Autodesk Inventor part; units mm, degrees
(part 4 of 16)
  spline S18 degree 3 poles (-31.6012, 101.0382) (-31.4716, 101.001) (-31.3425, 100.9618) (-31.2141, 100.9205) (-31.1447, 100.8982) (-31.0755, 100.8753) (-31.0064, 100.8518) (-30.9411, 100.8296) (-30.876, 100.8067) (-30.8111, 100.7833) (-30.7498, 100.7612) (-30.6887, 100.7385) (-30.6278, 100.7153) (-30.5706, 100.6935) (-30.5136, 100.6712) (-30.4567, 100.6484) (-30.4035, 100.627) (-30.3504, 100.6052) (-30.2976, 100.5829) (-30.2483, 100.5621) (-30.1992, 100.5408) (-30.1504, 100.5192) (-30.105, 100.4991) (-30.0599, 100.4786) (-30.0149, 100.4577) (-29.9734, 100.4384) (-29.9322, 100.4188) (-29.8911, 100.3988) (-29.8535, 100.3805) (-29.816, 100.3618) (-29.7787, 100.3429) (-29.7449, 100.3257) (-29.7113, 100.3082) (-29.6778, 100.2904) (-29.6477, 100.2744) (-29.6178, 100.2582) (-29.588, 100.2417) (-29.5487, 100.2198) (-29.5097, 100.1974) (-29.4708, 100.1747) (-29.4621, 100.1696) (-29.4535, 100.1645) (-29.4447, 100.1595) (-29.4362, 100.1546) (-29.4276, 100.1498) (-29.419, 100.1451) (-29.4105, 100.1404) (-29.4021, 100.1359) (-29.3935, 100.1314) (-29.3852, 100.127) (-29.3768, 100.1227) (-29.3684, 100.1184) (-29.3601, 100.1143) (-29.3518, 100.1102) (-29.3434, 100.1062) (-29.3352, 100.1023) (-29.3269, 100.0984) (-29.3186, 100.0947) (-29.3104, 100.091) (-29.3021, 100.0874) (-29.2938, 100.0839) (-29.2856, 100.0804) (-29.2774, 100.077) (-29.2691, 100.0737) (-29.2608, 100.0705) (-29.2525, 100.0674) (-29.2441, 100.0643) (-29.2357, 100.0613) (-29.2273, 100.0584) (-29.2189, 100.0556) (-29.2103, 100.0528) (-29.2017, 100.0501) (-29.1931, 100.0476) (-29.1843, 100.0451) (-29.1755, 100.0427) (-29.1666, 100.0404) (-29.1575, 100.0381) (-29.1483, 100.036) (-29.1391, 100.0341) (-29.1295, 100.0321) (-29.1199, 100.0303) (-29.1102, 100.0288) (-29.1, 100.0271) (-29.0898, 100.0257) (-29.0795, 100.0246) (-29.0685, 100.0235) (-29.0574, 100.0226) (-29.0464, 100.0221) (-29.0343, 100.0216) (-29.0223, 100.0214) (-29.0103, 100.0217) (-28.997, 100.0221) (-28.9837, 100.0229) (-28.9705, 100.0243) (-28.9558, 100.0259) (-28.9412, 100.0282) (-28.9266, 100.0312) (-28.9103, 100.0345) (-28.8942, 100.0387) (-28.8783, 100.0439) (-28.8605, 100.0497) (-28.8431, 100.0566) (-28.8262, 100.0646) (-28.8074, 100.0735) (-28.7893, 100.0838) (-28.7719, 100.0953) (-28.7531, 100.1078) (-28.7353, 100.1218) (-28.7189, 100.1373) (-28.7032, 100.1521) (-28.6889, 100.1682) (-28.6748, 100.1845) (-28.6053, 100.2653) (-28.5428, 100.3517) (-28.4763, 100.4349) (-28.4098, 100.518) (-28.3392, 100.5979) (-28.2756, 100.6835) (-28.2628, 100.7008) (-28.2502, 100.7183) (-28.2392, 100.7368) (-28.2277, 100.7562) (-28.218, 100.7767) (-28.2099, 100.7978) (-28.2024, 100.8172) (-28.1964, 100.8372) (-28.1918, 100.8574) (-28.1877, 100.8757) (-28.1848, 100.8942) (-28.183, 100.9129) (-28.1815, 100.9295) (-28.1809, 100.9461) (-28.1812, 100.9628) (-28.1815, 100.9776) (-28.1825, 100.9924) (-28.1842, 101.0071) (-28.1857, 101.0203) (-28.1878, 101.0334) (-28.1904, 101.0464) (-28.1927, 101.0582) (-28.1955, 101.07) (-28.1987, 101.0816) (-28.2016, 101.0923) (-28.2048, 101.1028) (-28.2084, 101.1133) (-28.2117, 101.1231) (-28.2153, 101.1328) (-28.2192, 101.1424) (-28.2228, 101.1515) (-28.2266, 101.1605) (-28.2307, 101.1694) (-28.2346, 101.178) (-28.2387, 101.1865) (-28.2429, 101.1949) (-28.247, 101.2031) (-28.2513, 101.2112) (-28.2558, 101.2192) (-28.2601, 101.227) (-28.2646, 101.2348) (-28.2692, 101.2425) (-28.2738, 101.2502) (-28.2784, 101.2578) (-28.2832, 101.2653) (-28.288, 101.2727) (-28.2929, 101.2802) (-28.2979, 101.2875) (-28.3029, 101.2949) (-28.308, 101.3022) (-28.3132, 101.3095) (-28.3185, 101.3168) (-28.3238, 101.3241) (-28.3292, 101.3313) (-28.3347, 101.3385) (-28.3402, 101.3458) (-28.3459, 101.3529) (-28.3516, 101.3602) (-28.3574, 101.3674) (-28.3633, 101.3746) (-28.3693, 101.3819) (-28.3753, 101.3891) (-28.3814, 101.3963) (-28.3877, 101.4037) (-28.394, 101.4109) (-28.4004, 101.4181) (-28.4069, 101.4255) (-28.4134, 101.4329) (-28.4201, 101.4401) (-28.4269, 101.4475) (-28.4338, 101.4549) (-28.4406, 101.4622) (-28.4713, 101.4951) (-28.5017, 101.5283) (-28.5317, 101.5619) (-28.5544, 101.5873) (-28.5767, 101.6129) (-28.5989, 101.6388) (-28.6236, 101.6675) (-28.6481, 101.6965) (-28.6723, 101.7258) (-28.699, 101.758) (-28.7254, 101.7904) (-28.7515, 101.8231) (-28.78, 101.8588) (-28.8082, 101.8948) (-28.8361, 101.931) (-28.8663, 101.9703) (-28.8962, 102.0098) (-28.9258, 102.0496) (-28.9577, 102.0926) (-28.9892, 102.1358) (-29.0203, 102.1793) (-29.0536, 102.226) (-29.0866, 102.2729) (-29.1191, 102.3202) (-29.1538, 102.3706) (-29.1881, 102.4214) (-29.222, 102.4724) (-29.2579, 102.5267) (-29.2934, 102.5814) (-29.3284, 102.6363) (-29.3655, 102.6945) (-29.4021, 102.753) (-29.4382, 102.8119) (-29.4763, 102.8741) (-29.5138, 102.9366) (-29.5508, 102.9994) (-29.6192, 103.1156) (-29.6857, 103.233) (-29.7505, 103.3512) knots 0 0 0 0 0.057795 0.057795 0.057795 0.089038 0.089038 0.089038 0.118617 0.118617 0.118617 0.14653 0.14653 0.14653 0.172778 0.172778 0.172778 0.19736 0.19736 0.19736 0.220277 0.220277 0.220277 0.241529 0.241529 0.241529 0.261115 0.261115 0.261115 0.279036 0.279036 0.279036 0.295292 0.295292 0.295292 0.309882 0.309882 0.309882 0.329164 0.329164 0.329164 0.333477 0.333477 0.333477 0.337694 0.337694 0.337694 0.34182 0.34182 0.34182 0.345864 0.345864 0.345864 0.349834 0.349834 0.349834 0.353742 0.353742 0.353742 0.3576 0.3576 0.3576 0.361424 0.361424 0.361424 0.365232 0.365232 0.365232 0.369048 0.369048 0.369048 0.372899 0.372899 0.372899 0.376819 0.376819 0.376819 0.380853 0.380853 0.380853 0.385052 0.385052 0.385052 0.389482 0.389482 0.389482 0.394225 0.394225 0.394225 0.399381 0.399381 0.399381 0.405067 0.405067 0.405067 0.411413 0.411413 0.411413 0.418548 0.418548 0.418548 0.426565 0.426565 0.426565 0.435472 0.435472 0.435472 0.445133 0.445133 0.445133 0.45436 0.45436 0.45436 0.5 0.5 0.5 0.54564 0.54564 0.54564 0.554867 0.554867 0.554867 0.564528 0.564528 0.564528 0.573435 0.573435 0.573435 0.581452 0.581452 0.581452 0.588587 0.588587 0.588587 0.594933 0.594933 0.594933 0.600619 0.600619 0.600619 0.605775 0.605775 0.605775 0.610518 0.610518 0.610518 0.614948 0.614948 0.614948 0.619147 0.619147 0.619147 0.623181 0.623181 0.623181 0.627101 0.627101 0.627101 0.630952 0.630952 0.630952 0.634768 0.634768 0.634768 0.638576 0.638576 0.638576 0.6424 0.6424 0.6424 0.646258 0.646258 0.646258 0.650166 0.650166 0.650166 0.654136 0.654136 0.654136 0.65818 0.65818 0.65818 0.662306 0.662306 0.662306 0.666523 0.666523 0.666523 0.670836 0.670836 0.670836 0.690118 0.690118 0.690118 0.704708 0.704708 0.704708 0.720964 0.720964 0.720964 0.738885 0.738885 0.738885 0.758471 0.758471 0.758471 0.779723 0.779723 0.779723 0.80264 0.80264 0.80264 0.827222 0.827222 0.827222 0.85347 0.85347 0.85347 0.881383 0.881383 0.881383 0.910962 0.910962 0.910962 0.942205 0.942205 0.942205 1 1 1 1
  arc A220 (-31.6012, 101.0382) -> (-32.2774, 100.0959) centre (0.0435, 77.6158) ccw
  spline S19 degree 3 poles (-33.8761, 97.6022) (-33.7433, 97.5786) (-33.6109, 97.5531) (-33.4789, 97.5256) (-33.4075, 97.5106) (-33.3363, 97.4951) (-33.2652, 97.4789) (-33.1979, 97.4636) (-33.1307, 97.4477) (-33.0637, 97.4312) (-33.0004, 97.4156) (-32.9373, 97.3995) (-32.8744, 97.3828) (-32.8152, 97.3671) (-32.7561, 97.3509) (-32.6972, 97.3341) (-32.642, 97.3184) (-32.587, 97.3022) (-32.5321, 97.2856) (-32.4809, 97.27) (-32.4299, 97.254) (-32.379, 97.2376) (-32.3318, 97.2223) (-32.2848, 97.2067) (-32.2379, 97.1906) (-32.1946, 97.1757) (-32.1515, 97.1605) (-32.1086, 97.1449) (-32.0692, 97.1307) (-32.0301, 97.1161) (-31.991, 97.1011) (-31.9556, 97.0875) (-31.9203, 97.0736) (-31.8851, 97.0594) (-31.8535, 97.0467) (-31.8221, 97.0337) (-31.7907, 97.0204) (-31.7493, 97.0028) (-31.7082, 96.9845) (-31.6672, 96.966) (-31.658, 96.9619) (-31.6489, 96.9577) (-31.6396, 96.9536) (-31.6306, 96.9497) (-31.6216, 96.9458) (-31.6125, 96.942) (-31.6036, 96.9382) (-31.5947, 96.9346) (-31.5858, 96.931) (-31.577, 96.9275) (-31.5682, 96.9241) (-31.5594, 96.9208) (-31.5507, 96.9175) (-31.542, 96.9143) (-31.5333, 96.9112) (-31.5247, 96.9082) (-31.5161, 96.9052) (-31.5074, 96.9024) (-31.4989, 96.8995) (-31.4903, 96.8968) (-31.4817, 96.8942) (-31.4731, 96.8916) (-31.4646, 96.8891) (-31.456, 96.8867) (-31.4474, 96.8844) (-31.4388, 96.8821) (-31.4302, 96.88) (-31.4215, 96.8778) (-31.4129, 96.8758) (-31.4042, 96.8739) (-31.3954, 96.872) (-31.3866, 96.8703) (-31.3777, 96.8687) (-31.3687, 96.8671) (-31.3597, 96.8656) (-31.3506, 96.8643) (-31.3413, 96.863) (-31.332, 96.8618) (-31.3226, 96.8609) (-31.3129, 96.8599) (-31.3031, 96.8591) (-31.2933, 96.8586) (-31.283, 96.858) (-31.2726, 96.8577) (-31.2623, 96.8577) (-31.2512, 96.8577) (-31.2402, 96.858) (-31.2291, 96.8587) (-31.2171, 96.8594) (-31.2051, 96.8605) (-31.1932, 96.8621) (-31.18, 96.8638) (-31.1669, 96.866) (-31.1539, 96.8688) (-31.1395, 96.8719) (-31.1251, 96.8757) (-31.111, 96.8802) (-31.0951, 96.8852) (-31.0795, 96.8911) (-31.0643, 96.8979) (-31.0472, 96.9055) (-31.0306, 96.9142) (-31.0146, 96.9239) (-30.9968, 96.9347) (-30.9799, 96.9469) (-30.9638, 96.9602) (-30.9465, 96.9746) (-30.9302, 96.9903) (-30.9155, 97.0074) (-30.9014, 97.0238) (-30.8889, 97.0413) (-30.8766, 97.059) (-30.8159, 97.1467) (-30.7628, 97.2391) (-30.7053, 97.3287) (-30.6479, 97.4184) (-30.586, 97.5052) (-30.5317, 97.5969) (-30.5207, 97.6155) (-30.5101, 97.6343) (-30.5011, 97.6538) (-30.4917, 97.6743) (-30.4841, 97.6957) (-30.4783, 97.7175) (-30.4729, 97.7376) (-30.469, 97.7581) (-30.4665, 97.7787) (-30.4644, 97.7973) (-30.4634, 97.8161) (-30.4636, 97.8348) (-30.4638, 97.8514) (-30.465, 97.8681) (-30.467, 97.8846) (-30.4689, 97.8993) (-30.4714, 97.9139) (-30.4746, 97.9284) (-30.4775, 97.9413) (-30.481, 97.9542) (-30.4849, 97.9668) (-30.4885, 97.9783) (-30.4924, 97.9897) (-30.4968, 98.0009) (-30.5008, 98.0112) (-30.5052, 98.0214) (-30.5098, 98.0315) (-30.5141, 98.0409) (-30.5187, 98.0501) (-30.5235, 98.0593) (-30.5281, 98.068) (-30.5329, 98.0765) (-30.5378, 98.085) (-30.5426, 98.0931) (-30.5476, 98.1011) (-30.5527, 98.109) (-30.5576, 98.1167) (-30.5627, 98.1243) (-30.568, 98.1318) (-30.5731, 98.1392) (-30.5784, 98.1464) (-30.5838, 98.1536) (-30.5891, 98.1607) (-30.5946, 98.1678) (-30.6001, 98.1748) (-30.6056, 98.1817) (-30.6113, 98.1886) (-30.617, 98.1954) (-30.6228, 98.2022) (-30.6286, 98.2089) (-30.6345, 98.2156) (-30.6405, 98.2223) (-30.6466, 98.229) (-30.6527, 98.2356) (-30.6589, 98.2423) (-30.6652, 98.2489) (-30.6716, 98.2554) (-30.678, 98.262) (-30.6845, 98.2686) (-30.6911, 98.2751) (-30.6978, 98.2818) (-30.7046, 98.2883) (-30.7115, 98.2948) (-30.7184, 98.3015) (-30.7255, 98.308) (-30.7326, 98.3146) (-30.7398, 98.3212) (-30.7471, 98.3278) (-30.7545, 98.3343) (-30.762, 98.341) (-30.7696, 98.3476) (-30.7772, 98.3542) (-30.8112, 98.3837) (-30.8449, 98.4135) (-30.8782, 98.4438) (-30.9034, 98.4667) (-30.9283, 98.4898) (-30.9531, 98.5132) (-30.9807, 98.5393) (-31.008, 98.5655) (-31.0352, 98.5921) (-31.0651, 98.6213) (-31.0947, 98.6508) (-31.1241, 98.6806) (-31.1562, 98.7131) (-31.188, 98.7459) (-31.2195, 98.779) (-31.2537, 98.8149) (-31.2876, 98.8512) (-31.3211, 98.8877) (-31.3573, 98.927) (-31.3932, 98.9667) (-31.4286, 99.0068) (-31.4667, 99.0497) (-31.5044, 99.0929) (-31.5417, 99.1365) (-31.5815, 99.1831) (-31.6209, 99.23) (-31.6599, 99.2772) (-31.7013, 99.3274) (-31.7423, 99.3781) (-31.7829, 99.429) (-31.8259, 99.483) (-31.8684, 99.5374) (-31.9104, 99.5922) (-31.9548, 99.65) (-31.9986, 99.7083) (-32.0419, 99.7669) (-32.1221, 99.8754) (-32.2006, 99.9851) (-32.2774, 100.0959) knots 0 0 0 0 0.057795 0.057795 0.057795 0.089038 0.089038 0.089038 0.118617 0.118617 0.118617 0.14653 0.14653 0.14653 0.172778 0.172778 0.172778 0.19736 0.19736 0.19736 0.220277 0.220277 0.220277 0.241529 0.241529 0.241529 0.261115 0.261115 0.261115 0.279036 0.279036 0.279036 0.295292 0.295292 0.295292 0.309882 0.309882 0.309882 0.329164 0.329164 0.329164 0.333477 0.333477 0.333477 0.337694 0.337694 0.337694 0.34182 0.34182 0.34182 0.345864 0.345864 0.345864 0.349834 0.349834 0.349834 0.353742 0.353742 0.353742 0.3576 0.3576 0.3576 0.361424 0.361424 0.361424 0.365232 0.365232 0.365232 0.369048 0.369048 0.369048 0.372899 0.372899 0.372899 0.376819 0.376819 0.376819 0.380853 0.380853 0.380853 0.385052 0.385052 0.385052 0.389482 0.389482 0.389482 0.394225 0.394225 0.394225 0.399381 0.399381 0.399381 0.405067 0.405067 0.405067 0.411413 0.411413 0.411413 0.418548 0.418548 0.418548 0.426565 0.426565 0.426565 0.435472 0.435472 0.435472 0.445133 0.445133 0.445133 0.45436 0.45436 0.45436 0.5 0.5 0.5 0.54564 0.54564 0.54564 0.554867 0.554867 0.554867 0.564528 0.564528 0.564528 0.573435 0.573435 0.573435 0.581452 0.581452 0.581452 0.588587 0.588587 0.588587 0.594933 0.594933 0.594933 0.600619 0.600619 0.600619 0.605775 0.605775 0.605775 0.610518 0.610518 0.610518 0.614948 0.614948 0.614948 0.619147 0.619147 0.619147 0.623181 0.623181 0.623181 0.627101 0.627101 0.627101 0.630952 0.630952 0.630952 0.634768 0.634768 0.634768 0.638576 0.638576 0.638576 0.6424 0.6424 0.6424 0.646258 0.646258 0.646258 0.650166 0.650166 0.650166 0.654136 0.654136 0.654136 0.65818 0.65818 0.65818 0.662306 0.662306 0.662306 0.666523 0.666523 0.666523 0.670836 0.670836 0.670836 0.690118 0.690118 0.690118 0.704708 0.704708 0.704708 0.720964 0.720964 0.720964 0.738885 0.738885 0.738885 0.758471 0.758471 0.758471 0.779723 0.779723 0.779723 0.80264 0.80264 0.80264 0.827222 0.827222 0.827222 0.85347 0.85347 0.85347 0.881383 0.881383 0.881383 0.910962 0.910962 0.910962 0.942205 0.942205 0.942205 1 1 1 1
  arc A221 (-33.8761, 97.6022) -> (-34.4501, 96.5943) centre (0.0435, 77.6158) ccw
  spline S20 degree 3 poles (-35.7795, 93.9471) (-35.6449, 93.9376) (-35.5105, 93.9261) (-35.3764, 93.9124) (-35.3038, 93.9051) (-35.2314, 93.8971) (-35.159, 93.8884) (-35.0904, 93.8802) (-35.022, 93.8714) (-34.9536, 93.862) (-34.8891, 93.8531) (-34.8246, 93.8437) (-34.7603, 93.8336) (-34.6997, 93.8242) (-34.6393, 93.8143) (-34.579, 93.8037) (-34.5225, 93.7939) (-34.466, 93.7836) (-34.4097, 93.7727) (-34.3572, 93.7626) (-34.3048, 93.7521) (-34.2524, 93.741) (-34.2039, 93.7308) (-34.1555, 93.7201) (-34.1071, 93.709) (-34.0626, 93.6988) (-34.0181, 93.6882) (-33.9738, 93.6772) (-33.9332, 93.6671) (-33.8927, 93.6566) (-33.8523, 93.6458) (-33.8156, 93.636) (-33.7791, 93.6259) (-33.7426, 93.6155) (-33.7099, 93.6061) (-33.6772, 93.5965) (-33.6447, 93.5865) (-33.6017, 93.5733) (-33.5588, 93.5595) (-33.5161, 93.5453) (-33.5066, 93.5422) (-33.497, 93.539) (-33.4874, 93.5359) (-33.4781, 93.5329) (-33.4687, 93.53) (-33.4593, 93.5271) (-33.45, 93.5244) (-33.4408, 93.5217) (-33.4315, 93.5191) (-33.4224, 93.5165) (-33.4133, 93.514) (-33.4042, 93.5116) (-33.3952, 93.5093) (-33.3863, 93.507) (-33.3772, 93.5049) (-33.3684, 93.5027) (-33.3595, 93.5007) (-33.3506, 93.4987) (-33.3418, 93.4968) (-33.333, 93.495) (-33.3241, 93.4933) (-33.3154, 93.4916) (-33.3066, 93.49) (-33.2978, 93.4886) (-33.289, 93.4871) (-33.2802, 93.4858) (-33.2714, 93.4845) (-33.2626, 93.4833) (-33.2538, 93.4822) (-33.2449, 93.4813) (-33.236, 93.4803) (-33.227, 93.4795) (-33.2181, 93.4788) (-33.2089, 93.4781) (-33.1998, 93.4776) (-33.1907, 93.4773) (-33.1813, 93.4769) (-33.1718, 93.4768) (-33.1624, 93.4768) (-33.1526, 93.4768) (-33.1428, 93.4771) (-33.1331, 93.4776) (-33.1227, 93.4781) (-33.1124, 93.4789) (-33.1021, 93.48) (-33.0911, 93.4811) (-33.0801, 93.4826) (-33.0692, 93.4844) (-33.0573, 93.4863) (-33.0455, 93.4887) (-33.0338, 93.4915) (-33.0209, 93.4946) (-33.0081, 93.4982) (-32.9955, 93.5023) (-32.9814, 93.5069) (-32.9676, 93.5122) (-32.954, 93.5181) (-32.9387, 93.5248) (-32.9238, 93.5323) (-32.9094, 93.5406) (-32.8932, 93.5499) (-32.8776, 93.5603) (-32.8627, 93.5717) (-32.8462, 93.5843) (-32.8306, 93.5981) (-32.816, 93.613) (-32.8002, 93.6292) (-32.7857, 93.6466) (-32.7729, 93.6651) (-32.7606, 93.6828) (-32.7499, 93.7016) (-32.7396, 93.7205) (-32.6884, 93.814) (-32.6452, 93.9115) (-32.5974, 94.0066) (-32.5497, 94.1018) (-32.4972, 94.1946) (-32.4528, 94.2915) (-32.4438, 94.3111) (-32.4352, 94.3309) (-32.4283, 94.3513) (-32.4211, 94.3726) (-32.4158, 94.3947) (-32.4123, 94.417) (-32.409, 94.4375) (-32.4073, 94.4583) (-32.407, 94.4791) (-32.4068, 94.4978) (-32.4078, 94.5166) (-32.41, 94.5352) (-32.4119, 94.5517) (-32.4148, 94.5681) (-32.4186, 94.5844) (-32.4219, 94.5988) (-32.426, 94.6131) (-32.4307, 94.6271) (-32.4349, 94.6397) (-32.4397, 94.6521) (-32.4449, 94.6643) (-32.4497, 94.6753) (-32.4548, 94.6862) (-32.4603, 94.6969) (-32.4654, 94.7068) (-32.4708, 94.7164) (-32.4764, 94.7259) (-32.4817, 94.7348) (-32.4873, 94.7436) (-32.493, 94.7522) (-32.4985, 94.7603) (-32.5041, 94.7683) (-32.5099, 94.7762) (-32.5155, 94.7838) (-32.5213, 94.7912) (-32.5272, 94.7986) (-32.5329, 94.8057) (-32.5388, 94.8127) (-32.5448, 94.8196) (-32.5507, 94.8264) (-32.5567, 94.8331) (-32.5628, 94.8397) (-32.5688, 94.8462) (-32.575, 94.8527) (-32.5812, 94.859) (-32.5875, 94.8653) (-32.5938, 94.8716) (-32.6002, 94.8777) (-32.6066, 94.8839) (-32.6132, 94.89) (-32.6197, 94.896) (-32.6264, 94.9021) (-32.6331, 94.9081) (-32.6399, 94.914) (-32.6468, 94.92) (-32.6537, 94.9259) (-32.6607, 94.9317) (-32.6678, 94.9377) (-32.675, 94.9435) (-32.6823, 94.9493) (-32.6896, 94.9552) (-32.6971, 94.961) (-32.7045, 94.9668) (-32.7122, 94.9727) (-32.7199, 94.9785) (-32.7276, 94.9842) (-32.7355, 94.9901) (-32.7434, 94.9959) (-32.7514, 95.0016) (-32.7596, 95.0074) (-32.7679, 95.0132) (-32.7761, 95.019) (-32.813, 95.0448) (-32.8497, 95.0709) (-32.8859, 95.0975) (-32.9134, 95.1176) (-32.9406, 95.1381) (-32.9677, 95.1587) (-32.9978, 95.1817) (-33.0278, 95.205) (-33.0575, 95.2285) (-33.0903, 95.2545) (-33.1229, 95.2808) (-33.1552, 95.3073) (-33.1905, 95.3363) (-33.2256, 95.3656) (-33.2604, 95.3952) (-33.2982, 95.4274) (-33.3356, 95.4598) (-33.3728, 95.4926) (-33.4129, 95.528) (-33.4527, 95.5638) (-33.4922, 95.5998) (-33.5345, 95.6385) (-33.5765, 95.6776) (-33.6182, 95.7171) (-33.6626, 95.7592) (-33.7067, 95.8017) (-33.7504, 95.8446) (-33.7969, 95.8903) (-33.843, 95.9363) (-33.8886, 95.9828) (-33.937, 96.032) (-33.985, 96.0816) (-34.0325, 96.1317) (-34.0827, 96.1846) (-34.1324, 96.238) (-34.1816, 96.2917) (-34.2727, 96.3912) (-34.3622, 96.4921) (-34.4501, 96.5943) knots 0 0 0 0 0.057795 0.057795 0.057795 0.089038 0.089038 0.089038 0.118617 0.118617 0.118617 0.14653 0.14653 0.14653 0.172778 0.172778 0.172778 0.19736 0.19736 0.19736 0.220277 0.220277 0.220277 0.241529 0.241529 0.241529 0.261115 0.261115 0.261115 0.279036 0.279036 0.279036 0.295292 0.295292 0.295292 0.309882 0.309882 0.309882 0.329164 0.329164 0.329164 0.333477 0.333477 0.333477 0.337694 0.337694 0.337694 0.34182 0.34182 0.34182 0.345864 0.345864 0.345864 0.349834 0.349834 0.349834 0.353742 0.353742 0.353742 0.3576 0.3576 0.3576 0.361424 0.361424 0.361424 0.365232 0.365232 0.365232 0.369048 0.369048 0.369048 0.372899 0.372899 0.372899 0.376819 0.376819 0.376819 0.380853 0.380853 0.380853 0.385052 0.385052 0.385052 0.389482 0.389482 0.389482 0.394225 0.394225 0.394225 0.399381 0.399381 0.399381 0.405067 0.405067 0.405067 0.411413 0.411413 0.411413 0.418548 0.418548 0.418548 0.426565 0.426565 0.426565 0.435472 0.435472 0.435472 0.445133 0.445133 0.445133 0.45436 0.45436 0.45436 0.5 0.5 0.5 0.54564 0.54564 0.54564 0.554867 0.554867 0.554867 0.564528 0.564528 0.564528 0.573435 0.573435 0.573435 0.581452 0.581452 0.581452 0.588587 0.588587 0.588587 0.594933 0.594933 0.594933 0.600619 0.600619 0.600619 0.605775 0.605775 0.605775 0.610518 0.610518 0.610518 0.614948 0.614948 0.614948 0.619147 0.619147 0.619147 0.623181 0.623181 0.623181 0.627101 0.627101 0.627101 0.630952 0.630952 0.630952 0.634768 0.634768 0.634768 0.638576 0.638576 0.638576 0.6424 0.6424 0.6424 0.646258 0.646258 0.646258 0.650166 0.650166 0.650166 0.654136 0.654136 0.654136 0.65818 0.65818 0.65818 0.662306 0.662306 0.662306 0.666523 0.666523 0.666523 0.670836 0.670836 0.670836 0.690118 0.690118 0.690118 0.704708 0.704708 0.704708 0.720964 0.720964 0.720964 0.738885 0.738885 0.738885 0.758471 0.758471 0.758471 0.779723 0.779723 0.779723 0.80264 0.80264 0.80264 0.827222 0.827222 0.827222 0.85347 0.85347 0.85347 0.881383 0.881383 0.881383 0.910962 0.910962 0.910962 0.942205 0.942205 0.942205 1 1 1 1
  arc A222 (-35.7795, 93.9471) -> (-36.245, 92.8848) centre (0.0435, 77.6158) ccw
  spline S21 degree 3 poles (-37.2903, 90.1131) (-37.1555, 90.1177) (-37.0207, 90.1203) (-36.8858, 90.1208) (-36.8129, 90.121) (-36.74, 90.1207) (-36.6671, 90.1196) (-36.5981, 90.1186) (-36.5291, 90.117) (-36.4601, 90.1148) (-36.395, 90.1127) (-36.3299, 90.1101) (-36.2648, 90.1068) (-36.2037, 90.1038) (-36.1425, 90.1002) (-36.0814, 90.096) (-36.0242, 90.0921) (-35.967, 90.0878) (-35.9098, 90.0829) (-35.8565, 90.0783) (-35.8033, 90.0733) (-35.7501, 90.0678) (-35.7008, 90.0627) (-35.6515, 90.0571) (-35.6023, 90.0511) (-35.5569, 90.0456) (-35.5116, 90.0397) (-35.4663, 90.0334) (-35.4249, 90.0276) (-35.3835, 90.0215) (-35.3422, 90.015) (-35.3047, 90.009) (-35.2673, 90.0028) (-35.23, 89.9962) (-35.1964, 89.9903) (-35.1629, 89.9842) (-35.1295, 89.9776) (-35.0854, 89.969) (-35.0413, 89.9597) (-34.9974, 89.9501) (-34.9875, 89.948) (-34.9777, 89.9458) (-34.9679, 89.9438) (-34.9582, 89.9417) (-34.9486, 89.9398) (-34.9389, 89.938) (-34.9295, 89.9362) (-34.92, 89.9345) (-34.9105, 89.9328) (-34.9012, 89.9312) (-34.8919, 89.9297) (-34.8825, 89.9283) (-34.8734, 89.9269) (-34.8642, 89.9256) (-34.855, 89.9244) (-34.846, 89.9232) (-34.8369, 89.9221) (-34.8279, 89.9211) (-34.8189, 89.9201) (-34.81, 89.9192) (-34.801, 89.9185) (-34.7921, 89.9177) (-34.7832, 89.917) (-34.7743, 89.9165) (-34.7654, 89.916) (-34.7565, 89.9155) (-34.7477, 89.9152) (-34.7388, 89.915) (-34.7299, 89.9148) (-34.721, 89.9148) (-34.712, 89.9147) (-34.703, 89.9149) (-34.694, 89.9151) (-34.6849, 89.9154) (-34.6757, 89.9158) (-34.6666, 89.9165) (-34.6572, 89.9171) (-34.6478, 89.9179) (-34.6385, 89.9189) (-34.6287, 89.92) (-34.619, 89.9213) (-34.6093, 89.9228) (-34.5991, 89.9244) (-34.5889, 89.9263) (-34.5788, 89.9284) (-34.568, 89.9307) (-34.5572, 89.9333) (-34.5465, 89.9362) (-34.5349, 89.9394) (-34.5235, 89.943) (-34.5121, 89.947) (-34.4996, 89.9514) (-34.4872, 89.9563) (-34.4751, 89.9618) (-34.4616, 89.9678) (-34.4484, 89.9745) (-34.4355, 89.9818) (-34.421, 89.99) (-34.407, 89.999) (-34.3935, 90.0088) (-34.3783, 90.0198) (-34.3639, 90.0318) (-34.3503, 90.0446) (-34.3351, 90.0589) (-34.3211, 90.0743) (-34.3082, 90.0906) (-34.2942, 90.1084) (-34.2815, 90.1272) (-34.2707, 90.1469) (-34.2604, 90.1658) (-34.2517, 90.1856) (-34.2434, 90.2055) (-34.2022, 90.3038) (-34.1695, 90.4053) (-34.1319, 90.5049) (-34.0944, 90.6045) (-34.0519, 90.7023) (-34.0179, 90.8034) (-34.011, 90.8238) (-34.0045, 90.8444) (-33.9998, 90.8654) (-33.9948, 90.8874) (-33.9919, 90.9098) (-33.9907, 90.9324) (-33.9896, 90.9532) (-33.99, 90.974) (-33.9919, 90.9947) (-33.9937, 91.0134) (-33.9966, 91.0319) (-34.0007, 91.0502) (-34.0044, 91.0664) (-34.009, 91.0825) (-34.0144, 91.0982) (-34.0193, 91.1122) (-34.0248, 91.126) (-34.031, 91.1394) (-34.0365, 91.1515) (-34.0425, 91.1633) (-34.049, 91.1749) (-34.0549, 91.1854) (-34.0611, 91.1957) (-34.0677, 91.2058) (-34.0738, 91.215) (-34.0802, 91.2241) (-34.0868, 91.233) (-34.093, 91.2412) (-34.0994, 91.2494) (-34.106, 91.2573) (-34.1123, 91.2648) (-34.1187, 91.2722) (-34.1253, 91.2794) (-34.1317, 91.2864) (-34.1382, 91.2932) (-34.1448, 91.2999) (-34.1513, 91.3064) (-34.1579, 91.3127) (-34.1645, 91.319) (-34.1711, 91.3251) (-34.1778, 91.3311) (-34.1845, 91.3371) (-34.1912, 91.3429) (-34.198, 91.3487) (-34.2049, 91.3543) (-34.2118, 91.36) (-34.2187, 91.3655) (-34.2257, 91.371) (-34.2328, 91.3764) (-34.2399, 91.3818) (-34.2471, 91.3871) (-34.2543, 91.3925) (-34.2617, 91.3977) (-34.269, 91.4029) (-34.2765, 91.4081) (-34.284, 91.4133) (-34.2916, 91.4184) (-34.2993, 91.4235) (-34.307, 91.4286) (-34.3148, 91.4336) (-34.3228, 91.4387) (-34.3308, 91.4437) (-34.3388, 91.4486) (-34.347, 91.4537) (-34.3553, 91.4586) (-34.3636, 91.4635) (-34.372, 91.4685) (-34.3805, 91.4735) (-34.3891, 91.4783) (-34.3979, 91.4833) (-34.4067, 91.4882) (-34.4155, 91.493) (-34.4548, 91.5148) (-34.494, 91.537) (-34.5329, 91.5596) (-34.5623, 91.5768) (-34.5915, 91.5943) (-34.6206, 91.612) (-34.653, 91.6317) (-34.6852, 91.6518) (-34.7172, 91.6721) (-34.7526, 91.6944) (-34.7877, 91.7172) (-34.8226, 91.7402) (-34.8608, 91.7653) (-34.8987, 91.7908) (-34.9364, 91.8166) (-34.9773, 91.8446) (-35.018, 91.873) (-35.0584, 91.9018) (-35.102, 91.9327) (-35.1453, 91.9641) (-35.1883, 91.9959) (-35.2345, 92.03) (-35.2803, 92.0644) (-35.3259, 92.0993) (-35.3745, 92.1366) (-35.4228, 92.1743) (-35.4707, 92.2124) (-35.5217, 92.2529) (-35.5724, 92.2939) (-35.6226, 92.3353) (-35.6759, 92.3792) (-35.7288, 92.4235) (-35.7813, 92.4684) (-35.8367, 92.5157) (-35.8917, 92.5636) (-35.9463, 92.6119) (-36.0473, 92.7013) (-36.1468, 92.7924) (-36.245, 92.8848) knots 0 0 0 0 0.057795 0.057795 0.057795 0.089038 0.089038 0.089038 0.118617 0.118617 0.118617 0.14653 0.14653 0.14653 0.172778 0.172778 0.172778 0.19736 0.19736 0.19736 0.220277 0.220277 0.220277 0.241529 0.241529 0.241529 0.261115 0.261115 0.261115 0.279036 0.279036 0.279036 0.295292 0.295292 0.295292 0.309882 0.309882 0.309882 0.329164 0.329164 0.329164 0.333477 0.333477 0.333477 0.337694 0.337694 0.337694 0.34182 0.34182 0.34182 0.345864 0.345864 0.345864 0.349834 0.349834 0.349834 0.353742 0.353742 0.353742 0.3576 0.3576 0.3576 0.361424 0.361424 0.361424 0.365232 0.365232 0.365232 0.369048 0.369048 0.369048 0.372899 0.372899 0.372899 0.376819 0.376819 0.376819 0.380853 0.380853 0.380853 0.385052 0.385052 0.385052 0.389482 0.389482 0.389482 0.394225 0.394225 0.394225 0.399381 0.399381 0.399381 0.405067 0.405067 0.405067 0.411413 0.411413 0.411413 0.418548 0.418548 0.418548 0.426565 0.426565 0.426565 0.435472 0.435472 0.435472 0.445133 0.445133 0.445133 0.45436 0.45436 0.45436 0.5 0.5 0.5 0.54564 0.54564 0.54564 0.554867 0.554867 0.554867 0.564528 0.564528 0.564528 0.573435 0.573435 0.573435 0.581452 0.581452 0.581452 0.588587 0.588587 0.588587 0.594933 0.594933 0.594933 0.600619 0.600619 0.600619 0.605775 0.605775 0.605775 0.610518 0.610518 0.610518 0.614948 0.614948 0.614948 0.619147 0.619147 0.619147 0.623181 0.623181 0.623181 0.627101 0.627101 0.627101 0.630952 0.630952 0.630952 0.634768 0.634768 0.634768 0.638576 0.638576 0.638576 0.6424 0.6424 0.6424 0.646258 0.646258 0.646258 0.650166 0.650166 0.650166 0.654136 0.654136 0.654136 0.65818 0.65818 0.65818 0.662306 0.662306 0.662306 0.666523 0.666523 0.666523 0.670836 0.670836 0.670836 0.690118 0.690118 0.690118 0.704708 0.704708 0.704708 0.720964 0.720964 0.720964 0.738885 0.738885 0.738885 0.758471 0.758471 0.758471 0.779723 0.779723 0.779723 0.80264 0.80264 0.80264 0.827222 0.827222 0.827222 0.85347 0.85347 0.85347 0.881383 0.881383 0.881383 0.910962 0.910962 0.910962 0.942205 0.942205 0.942205 1 1 1 1
  arc A223 (-37.2903, 90.1131) -> (-37.6422, 89.008) centre (0.0435, 77.6158) ccw
  spline S22 degree 3 poles (-38.3921, 86.1422) (-38.2586, 86.1609) (-38.1247, 86.1776) (-37.9906, 86.1921) (-37.9182, 86.2) (-37.8456, 86.2072) (-37.773, 86.2138) (-37.7042, 86.22) (-37.6355, 86.2257) (-37.5666, 86.2307) (-37.5016, 86.2354) (-37.4366, 86.2396) (-37.3716, 86.2431) (-37.3104, 86.2465) (-37.2493, 86.2493) (-37.1881, 86.2516) (-37.1307, 86.2537) (-37.0734, 86.2553) (-37.016, 86.2564) (-36.9626, 86.2575) (-36.9091, 86.258) (-36.8556, 86.2581) (-36.806, 86.2582) (-36.7564, 86.2578) (-36.7068, 86.257) (-36.6611, 86.2563) (-36.6154, 86.2551) (-36.5698, 86.2536) (-36.528, 86.2522) (-36.4862, 86.2504) (-36.4444, 86.2482) (-36.4065, 86.2462) (-36.3687, 86.244) (-36.3308, 86.2413) (-36.2969, 86.239) (-36.2629, 86.2363) (-36.229, 86.2333) (-36.1842, 86.2294) (-36.1394, 86.2248) (-36.0947, 86.2198) (-36.0847, 86.2187) (-36.0747, 86.2176) (-36.0647, 86.2165) (-36.0549, 86.2155) (-36.0451, 86.2146) (-36.0353, 86.2138) (-36.0257, 86.213) (-36.0161, 86.2123) (-36.0065, 86.2117) (-35.9971, 86.2111) (-35.9877, 86.2105) (-35.9782, 86.2101) (-35.969, 86.2097) (-35.9597, 86.2093) (-35.9505, 86.2091) (-35.9413, 86.2088) (-35.9322, 86.2087) (-35.9231, 86.2086) (-35.9141, 86.2086) (-35.9051, 86.2087) (-35.8961, 86.2088) (-35.8872, 86.209) (-35.8783, 86.2093) (-35.8693, 86.2097) (-35.8605, 86.2101) (-35.8516, 86.2106) (-35.8427, 86.2112) (-35.8338, 86.2118) (-35.825, 86.2126) (-35.8161, 86.2135) (-35.8072, 86.2144) (-35.7982, 86.2155) (-35.7893, 86.2167) (-35.7803, 86.2179) (-35.7712, 86.2193) (-35.7622, 86.2209) (-35.7529, 86.2225) (-35.7437, 86.2243) (-35.7345, 86.2263) (-35.7249, 86.2284) (-35.7154, 86.2307) (-35.7059, 86.2332) (-35.6959, 86.2358) (-35.686, 86.2387) (-35.6762, 86.2419) (-35.6656, 86.2453) (-35.6552, 86.249) (-35.6449, 86.2531) (-35.6337, 86.2575) (-35.6226, 86.2623) (-35.6118, 86.2674) (-35.5998, 86.2731) (-35.588, 86.2793) (-35.5765, 86.286) (-35.5637, 86.2934) (-35.5513, 86.3014) (-35.5392, 86.31) (-35.5257, 86.3197) (-35.5126, 86.3302) (-35.5003, 86.3413) (-35.4863, 86.3538) (-35.4732, 86.3672) (-35.461, 86.3814) (-35.4475, 86.3972) (-35.4351, 86.414) (-35.424, 86.4316) (-35.4119, 86.4507) (-35.4013, 86.4707) (-35.3926, 86.4915) (-35.3843, 86.5114) (-35.3777, 86.5319) (-35.3715, 86.5526) (-35.3409, 86.6547) (-35.319, 86.759) (-35.292, 86.862) (-35.2651, 86.965) (-35.2331, 87.0667) (-35.2098, 87.1707) (-35.2051, 87.1918) (-35.2007, 87.2129) (-35.1982, 87.2343) (-35.1956, 87.2567) (-35.195, 87.2793) (-35.1962, 87.3019) (-35.1973, 87.3227) (-35.1999, 87.3434) (-35.204, 87.3638) (-35.2076, 87.3821) (-35.2125, 87.4002) (-35.2185, 87.418) (-35.2239, 87.4338) (-35.2301, 87.4492) (-35.2372, 87.4643) (-35.2435, 87.4777) (-35.2504, 87.4908) (-35.2579, 87.5036) (-35.2647, 87.515) (-35.2719, 87.5262) (-35.2796, 87.537) (-35.2865, 87.5468) (-35.2938, 87.5564) (-35.3014, 87.5657) (-35.3084, 87.5743) (-35.3157, 87.5826) (-35.3232, 87.5908) (-35.3302, 87.5984) (-35.3375, 87.6058) (-35.3449, 87.613) (-35.3519, 87.6198) (-35.3591, 87.6265) (-35.3664, 87.633) (-35.3735, 87.6392) (-35.3806, 87.6453) (-35.3879, 87.6513) (-35.395, 87.657) (-35.4022, 87.6627) (-35.4095, 87.6682) (-35.4167, 87.6736) (-35.424, 87.6789) (-35.4313, 87.6841) (-35.4386, 87.6892) (-35.4459, 87.6942) (-35.4534, 87.6991) (-35.4608, 87.704) (-35.4683, 87.7088) (-35.4758, 87.7135) (-35.4834, 87.7182) (-35.491, 87.7228) (-35.4987, 87.7273) (-35.5065, 87.7319) (-35.5143, 87.7364) (-35.5222, 87.7407) (-35.5302, 87.7452) (-35.5382, 87.7495) (-35.5463, 87.7538) (-35.5544, 87.7581) (-35.5627, 87.7623) (-35.571, 87.7665) (-35.5794, 87.7707) (-35.5879, 87.7749) (-35.5964, 87.7789) (-35.6051, 87.7831) (-35.6138, 87.7872) (-35.6226, 87.7912) (-35.6315, 87.7953) (-35.6405, 87.7993) (-35.6495, 87.8032) (-35.6587, 87.8072) (-35.668, 87.8111) (-35.6773, 87.8151) (-35.7187, 87.8326) (-35.76, 87.8506) (-35.801, 87.869) (-35.832, 87.883) (-35.8629, 87.8974) (-35.8937, 87.912) (-35.928, 87.9282) (-35.9621, 87.9447) (-35.9961, 87.9616) (-36.0336, 87.9801) (-36.0709, 87.9991) (-36.108, 88.0183) (-36.1486, 88.0393) (-36.189, 88.0607) (-36.2292, 88.0824) (-36.2728, 88.106) (-36.3162, 88.13) (-36.3594, 88.1543) (-36.406, 88.1806) (-36.4524, 88.2073) (-36.4985, 88.2344) (-36.5479, 88.2634) (-36.5971, 88.2929) (-36.6461, 88.3229) (-36.6983, 88.3548) (-36.7503, 88.3873) (-36.8019, 88.4201) (-36.8569, 88.4551) (-36.9115, 88.4906) (-36.9659, 88.5265) (-37.0234, 88.5646) (-37.0806, 88.6032) (-37.1375, 88.6423) (-37.1976, 88.6836) (-37.2573, 88.7255) (-37.3167, 88.7678) (-37.4264, 88.8462) (-37.5349, 88.9263) (-37.6422, 89.008) knots 0 0 0 0 0.057795 0.057795 0.057795 0.089038 0.089038 0.089038 0.118617 0.118617 0.118617 0.14653 0.14653 0.14653 0.172778 0.172778 0.172778 0.19736 0.19736 0.19736 0.220277 0.220277 0.220277 0.241529 0.241529 0.241529 0.261115 0.261115 0.261115 0.279036 0.279036 0.279036 0.295292 0.295292 0.295292 0.309882 0.309882 0.309882 0.329164 0.329164 0.329164 0.333477 0.333477 0.333477 0.337694 0.337694 0.337694 0.34182 0.34182 0.34182 0.345864 0.345864 0.345864 0.349834 0.349834 0.349834 0.353742 0.353742 0.353742 0.3576 0.3576 0.3576 0.361424 0.361424 0.361424 0.365232 0.365232 0.365232 0.369048 0.369048 0.369048 0.372899 0.372899 0.372899 0.376819 0.376819 0.376819 0.380853 0.380853 0.380853 0.385052 0.385052 0.385052 0.389482 0.389482 0.389482 0.394225 0.394225 0.394225 0.399381 0.399381 0.399381 0.405067 0.405067 0.405067 0.411413 0.411413 0.411413 0.418548 0.418548 0.418548 0.426565 0.426565 0.426565 0.435472 0.435472 0.435472 0.445133 0.445133 0.445133 0.45436 0.45436 0.45436 0.5 0.5 0.5 0.54564 0.54564 0.54564 0.554867 0.554867 0.554867 0.564528 0.564528 0.564528 0.573435 0.573435 0.573435 0.581452 0.581452 0.581452 0.588587 0.588587 0.588587 0.594933 0.594933 0.594933 0.600619 0.600619 0.600619 0.605775 0.605775 0.605775 0.610518 0.610518 0.610518 0.614948 0.614948 0.614948 0.619147 0.619147 0.619147 0.623181 0.623181 0.623181 0.627101 0.627101 0.627101 0.630952 0.630952 0.630952 0.634768 0.634768 0.634768 0.638576 0.638576 0.638576 0.6424 0.6424 0.6424 0.646258 0.646258 0.646258 0.650166 0.650166 0.650166 0.654136 0.654136 0.654136 0.65818 0.65818 0.65818 0.662306 0.662306 0.662306 0.666523 0.666523 0.666523 0.670836 0.670836 0.670836 0.690118 0.690118 0.690118 0.704708 0.704708 0.704708 0.720964 0.720964 0.720964 0.738885 0.738885 0.738885 0.758471 0.758471 0.758471 0.779723 0.779723 0.779723 0.80264 0.80264 0.80264 0.827222 0.827222 0.827222 0.85347 0.85347 0.85347 0.881383 0.881383 0.881383 0.910962 0.910962 0.910962 0.942205 0.942205 0.942205 1 1 1 1
  arc A224 (-38.3921, 86.1422) -> (-38.6266, 85.0063) centre (0.0435, 77.6158) ccw
  spline S23 degree 3 poles (-39.0728, 82.0779) (-38.9419, 82.1104) (-38.8106, 82.141) (-38.6788, 82.1695) (-38.6075, 82.1849) (-38.5361, 82.1997) (-38.4646, 82.2138) (-38.3969, 82.2272) (-38.329, 82.24) (-38.2611, 82.2522) (-38.197, 82.2636) (-38.1328, 82.2746) (-38.0684, 82.2849) (-38.008, 82.2947) (-37.9474, 82.3039) (-37.8868, 82.3125) (-37.83, 82.3206) (-37.7731, 82.3282) (-37.7162, 82.3353) (-37.6631, 82.3419) (-37.61, 82.3481) (-37.5568, 82.3538) (-37.5075, 82.359) (-37.4582, 82.3639) (-37.4088, 82.3682) (-37.3632, 82.3723) (-37.3177, 82.3759) (-37.2721, 82.3791) (-37.2304, 82.3821) (-37.1886, 82.3847) (-37.1469, 82.3869) (-37.109, 82.3889) (-37.0711, 82.3906) (-37.0332, 82.3919) (-36.9992, 82.3931) (-36.9651, 82.3941) (-36.9311, 82.3946) (-36.8861, 82.3954) (-36.8411, 82.3955) (-36.7961, 82.3952) (-36.786, 82.3951) (-36.776, 82.3951) (-36.7659, 82.3951) (-36.7561, 82.3951) (-36.7462, 82.3953) (-36.7364, 82.3955) (-36.7268, 82.3957) (-36.7171, 82.396) (-36.7075, 82.3963) (-36.6981, 82.3967) (-36.6887, 82.3972) (-36.6792, 82.3977) (-36.67, 82.3983) (-36.6608, 82.3989) (-36.6515, 82.3996) (-36.6424, 82.4003) (-36.6333, 82.4011) (-36.6243, 82.402) (-36.6153, 82.4029) (-36.6064, 82.4039) (-36.5974, 82.405) (-36.5886, 82.4061) (-36.5797, 82.4074) (-36.5709, 82.4087) (-36.5621, 82.41) (-36.5533, 82.4114) (-36.5446, 82.413) (-36.5358, 82.4145) (-36.5271, 82.4162) (-36.5184, 82.4181) (-36.5096, 82.4199) (-36.5008, 82.4219) (-36.4921, 82.424) (-36.4832, 82.4262) (-36.4743, 82.4285) (-36.4655, 82.431) (-36.4565, 82.4336) (-36.4475, 82.4364) (-36.4385, 82.4393) (-36.4292, 82.4424) (-36.42, 82.4456) (-36.4108, 82.4491) (-36.4012, 82.4528) (-36.3916, 82.4568) (-36.3822, 82.4609) (-36.3721, 82.4654) (-36.3621, 82.4702) (-36.3522, 82.4753) (-36.3416, 82.4809) (-36.3311, 82.4868) (-36.3208, 82.493) (-36.3095, 82.5) (-36.2984, 82.5073) (-36.2877, 82.5151) (-36.2757, 82.5239) (-36.2642, 82.5332) (-36.2531, 82.543) (-36.2406, 82.5541) (-36.2288, 82.5658) (-36.2176, 82.5782) (-36.2051, 82.5921) (-36.1934, 82.6068) (-36.1828, 82.6222) (-36.171, 82.6393) (-36.1604, 82.6573) (-36.1512, 82.6759) (-36.1412, 82.6962) (-36.1327, 82.7172) (-36.1262, 82.7388) (-36.1201, 82.7594) (-36.1157, 82.7805) (-36.1117, 82.8017) (-36.0919, 82.9065) (-36.081, 83.0125) (-36.0649, 83.1178) (-36.0489, 83.223) (-36.0277, 83.3275) (-36.0154, 83.4334) (-36.0129, 83.4548) (-36.0108, 83.4763) (-36.0106, 83.4978) (-36.0103, 83.5204) (-36.0121, 83.543) (-36.0157, 83.5653) (-36.0189, 83.5858) (-36.0236, 83.6061) (-36.0298, 83.626) (-36.0354, 83.6439) (-36.0421, 83.6614) (-36.05, 83.6784) (-36.0569, 83.6935) (-36.0647, 83.7083) (-36.0733, 83.7225) (-36.081, 83.7352) (-36.0893, 83.7475) (-36.0981, 83.7594) (-36.106, 83.7701) (-36.1144, 83.7804) (-36.1231, 83.7904) (-36.131, 83.7994) (-36.1393, 83.8082) (-36.1478, 83.8167) (-36.1557, 83.8245) (-36.1638, 83.832) (-36.1721, 83.8393) (-36.1799, 83.8461) (-36.1879, 83.8527) (-36.196, 83.8591) (-36.2037, 83.8652) (-36.2115, 83.8711) (-36.2195, 83.8768) (-36.2272, 83.8822) (-36.2349, 83.8875) (-36.2428, 83.8927) (-36.2505, 83.8977) (-36.2582, 83.9026) (-36.2661, 83.9073) (-36.2738, 83.9119) (-36.2815, 83.9164) (-36.2894, 83.9208) (-36.2972, 83.9251) (-36.305, 83.9294) (-36.3129, 83.9335) (-36.3208, 83.9376) (-36.3288, 83.9415) (-36.3367, 83.9454) (-36.3448, 83.9493) (-36.3529, 83.9531) (-36.361, 83.9568) (-36.3692, 83.9605) (-36.3774, 83.9641) (-36.3857, 83.9676) (-36.3941, 83.9712) (-36.4025, 83.9747) (-36.411, 83.9781) (-36.4196, 83.9815) (-36.4282, 83.9849) (-36.4369, 83.9881) (-36.4457, 83.9915) (-36.4546, 83.9947) (-36.4635, 83.9979) (-36.4726, 84.0011) (-36.4817, 84.0042) (-36.4908, 84.0073) (-36.5001, 84.0104) (-36.5095, 84.0135) (-36.5189, 84.0165) (-36.5285, 84.0195) (-36.5381, 84.0224) (-36.5477, 84.0254) (-36.5907, 84.0385) (-36.6337, 84.052) (-36.6764, 84.0661) (-36.7087, 84.0768) (-36.7409, 84.0878) (-36.7731, 84.0991) (-36.8089, 84.1117) (-36.8445, 84.1245) (-36.8801, 84.1377) (-36.9193, 84.1523) (-36.9584, 84.1672) (-36.9973, 84.1824) (-37.0399, 84.1991) (-37.0823, 84.2162) (-37.1245, 84.2336) (-37.1704, 84.2525) (-37.2161, 84.2718) (-37.2616, 84.2915) (-37.3107, 84.3127) (-37.3595, 84.3344) (-37.4082, 84.3565) (-37.4605, 84.3803) (-37.5125, 84.4045) (-37.5643, 84.4291) (-37.6196, 84.4554) (-37.6746, 84.4823) (-37.7295, 84.5096) (-37.7878, 84.5386) (-37.8458, 84.5682) (-37.9036, 84.5982) (-37.9648, 84.6301) (-38.0258, 84.6625) (-38.0864, 84.6954) (-38.1505, 84.7302) (-38.2143, 84.7656) (-38.2777, 84.8015) (-38.3951, 84.868) (-38.5113, 84.9363) (-38.6266, 85.0063) knots 0 0 0 0 0.057795 0.057795 0.057795 0.089038 0.089038 0.089038 0.118617 0.118617 0.118617 0.14653 0.14653 0.14653 0.172778 0.172778 0.172778 0.19736 0.19736 0.19736 0.220277 0.220277 0.220277 0.241529 0.241529 0.241529 0.261115 0.261115 0.261115 0.279036 0.279036 0.279036 0.295292 0.295292 0.295292 0.309882 0.309882 0.309882 0.329164 0.329164 0.329164 0.333477 0.333477 0.333477 0.337694 0.337694 0.337694 0.34182 0.34182 0.34182 0.345864 0.345864 0.345864 0.349834 0.349834 0.349834 0.353742 0.353742 0.353742 0.3576 0.3576 0.3576 0.361424 0.361424 0.361424 0.365232 0.365232 0.365232 0.369048 0.369048 0.369048 0.372899 0.372899 0.372899 0.376819 0.376819 0.376819 0.380853 0.380853 0.380853 0.385052 0.385052 0.385052 0.389482 0.389482 0.389482 0.394225 0.394225 0.394225 0.399381 0.399381 0.399381 0.405067 0.405067 0.405067 0.411413 0.411413 0.411413 0.418548 0.418548 0.418548 0.426565 0.426565 0.426565 0.435472 0.435472 0.435472 0.445133 0.445133 0.445133 0.45436 0.45436 0.45436 0.5 0.5 0.5 0.54564 0.54564 0.54564 0.554867 0.554867 0.554867 0.564528 0.564528 0.564528 0.573435 0.573435 0.573435 0.581452 0.581452 0.581452 0.588587 0.588587 0.588587 0.594933 0.594933 0.594933 0.600619 0.600619 0.600619 0.605775 0.605775 0.605775 0.610518 0.610518 0.610518 0.614948 0.614948 0.614948 0.619147 0.619147 0.619147 0.623181 0.623181 0.623181 0.627101 0.627101 0.627101 0.630952 0.630952 0.630952 0.634768 0.634768 0.634768 0.638576 0.638576 0.638576 0.6424 0.6424 0.6424 0.646258 0.646258 0.646258 0.650166 0.650166 0.650166 0.654136 0.654136 0.654136 0.65818 0.65818 0.65818 0.662306 0.662306 0.662306 0.666523 0.666523 0.666523 0.670836 0.670836 0.670836 0.690118 0.690118 0.690118 0.704708 0.704708 0.704708 0.720964 0.720964 0.720964 0.738885 0.738885 0.738885 0.758471 0.758471 0.758471 0.779723 0.779723 0.779723 0.80264 0.80264 0.80264 0.827222 0.827222 0.827222 0.85347 0.85347 0.85347 0.881383 0.881383 0.881383 0.910962 0.910962 0.910962 0.942205 0.942205 0.942205 1 1 1 1
  arc A225 (-39.0728, 82.0779) -> (-39.1873, 80.9237) centre (0.0435, 77.6158) ccw
  spline S24 degree 3 poles (-39.325, 77.9647) (-39.1982, 78.0107) (-39.0707, 78.0549) (-38.9426, 78.097) (-38.8734, 78.1197) (-38.8039, 78.1419) (-38.7342, 78.1634) (-38.6683, 78.1838) (-38.6022, 78.2036) (-38.5359, 78.2228) (-38.4733, 78.241) (-38.4106, 78.2586) (-38.3477, 78.2756) (-38.2886, 78.2916) (-38.2293, 78.3071) (-38.1699, 78.322) (-38.1143, 78.336) (-38.0586, 78.3495) (-38.0027, 78.3625) (-37.9506, 78.3746) (-37.8984, 78.3863) (-37.8461, 78.3975) (-37.7976, 78.4079) (-37.749, 78.4179) (-37.7004, 78.4274) (-37.6555, 78.4361) (-37.6106, 78.4445) (-37.5656, 78.4525) (-37.5244, 78.4598) (-37.4832, 78.4668) (-37.4419, 78.4733) (-37.4044, 78.4793) (-37.3669, 78.4849) (-37.3293, 78.4902) (-37.2956, 78.4949) (-37.2619, 78.4994) (-37.2281, 78.5035) (-37.1834, 78.509) (-37.1387, 78.5138) (-37.0939, 78.5182) (-37.0839, 78.5192) (-37.0738, 78.5202) (-37.0638, 78.5213) (-37.0541, 78.5223) (-37.0443, 78.5235) (-37.0345, 78.5247) (-37.025, 78.526) (-37.0154, 78.5272) (-37.0059, 78.5286) (-36.9966, 78.53) (-36.9872, 78.5314) (-36.9779, 78.5329) (-36.9688, 78.5345) (-36.9597, 78.536) (-36.9505, 78.5377) (-36.9416, 78.5394) (-36.9326, 78.5411) (-36.9237, 78.543) (-36.9149, 78.5448) (-36.9061, 78.5468) (-36.8973, 78.5488) (-36.8886, 78.5508) (-36.88, 78.5529) (-36.8713, 78.5552) (-36.8627, 78.5574) (-36.8541, 78.5597) (-36.8456, 78.5622) (-36.8371, 78.5647) (-36.8285, 78.5673) (-36.8201, 78.57) (-36.8115, 78.5728) (-36.803, 78.5756) (-36.7945, 78.5787) (-36.7859, 78.5818) (-36.7774, 78.585) (-36.7689, 78.5884) (-36.7601, 78.5919) (-36.7515, 78.5956) (-36.7429, 78.5995) (-36.734, 78.6035) (-36.7251, 78.6077) (-36.7164, 78.6121) (-36.7071, 78.6168) (-36.698, 78.6217) (-36.6891, 78.6269) (-36.6795, 78.6324) (-36.6701, 78.6382) (-36.6608, 78.6443) (-36.6508, 78.6509) (-36.641, 78.6579) (-36.6314, 78.6652) (-36.6209, 78.6733) (-36.6106, 78.6818) (-36.6008, 78.6907) (-36.5898, 78.7006) (-36.5793, 78.711) (-36.5693, 78.722) (-36.558, 78.7343) (-36.5475, 78.7472) (-36.5377, 78.7607) (-36.5267, 78.7758) (-36.5166, 78.7916) (-36.5076, 78.8081) (-36.4977, 78.8263) (-36.4891, 78.8453) (-36.4818, 78.8648) (-36.474, 78.886) (-36.4678, 78.9078) (-36.4636, 78.93) (-36.4596, 78.9511) (-36.4575, 78.9726) (-36.4557, 78.9941) (-36.4469, 79.1003) (-36.4472, 79.2069) (-36.4422, 79.3133) (-36.4373, 79.4196) (-36.4271, 79.5258) (-36.426, 79.6324) (-36.4258, 79.6539) (-36.4259, 79.6755) (-36.4279, 79.6969) (-36.43, 79.7194) (-36.4342, 79.7417) (-36.44, 79.7635) (-36.4454, 79.7836) (-36.4522, 79.8033) (-36.4605, 79.8224) (-36.4679, 79.8396) (-36.4764, 79.8563) (-36.486, 79.8724) (-36.4945, 79.8867) (-36.5038, 79.9005) (-36.5138, 79.9138) (-36.5228, 79.9257) (-36.5323, 79.937) (-36.5423, 79.9479) (-36.5513, 79.9577) (-36.5607, 79.9671) (-36.5704, 79.9761) (-36.5792, 79.9843) (-36.5884, 79.9921) (-36.5978, 79.9997) (-36.6064, 80.0066) (-36.6152, 80.0133) (-36.6243, 80.0196) (-36.6327, 80.0256) (-36.6413, 80.0313) (-36.6501, 80.0369) (-36.6584, 80.0421) (-36.6668, 80.0471) (-36.6753, 80.0519) (-36.6835, 80.0566) (-36.6918, 80.0611) (-36.7002, 80.0654) (-36.7083, 80.0695) (-36.7165, 80.0736) (-36.7248, 80.0774) (-36.7329, 80.0812) (-36.7412, 80.0849) (-36.7494, 80.0884) (-36.7576, 80.0919) (-36.7658, 80.0953) (-36.7741, 80.0986) (-36.7824, 80.1018) (-36.7907, 80.1049) (-36.7991, 80.108) (-36.8075, 80.111) (-36.8159, 80.1139) (-36.8244, 80.1167) (-36.8329, 80.1196) (-36.8415, 80.1223) (-36.8501, 80.125) (-36.8588, 80.1276) (-36.8676, 80.1302) (-36.8763, 80.1327) (-36.8853, 80.1352) (-36.8942, 80.1376) (-36.9032, 80.14) (-36.9123, 80.1424) (-36.9214, 80.1447) (-36.9306, 80.1469) (-36.94, 80.1492) (-36.9494, 80.1513) (-36.9588, 80.1534) (-36.9684, 80.1556) (-36.978, 80.1576) (-36.9876, 80.1596) (-36.9975, 80.1616) (-37.0074, 80.1635) (-37.0172, 80.1654) (-37.0614, 80.174) (-37.1055, 80.1829) (-37.1495, 80.1925) (-37.1827, 80.1997) (-37.2159, 80.2073) (-37.2491, 80.2152) (-37.286, 80.224) (-37.3228, 80.233) (-37.3596, 80.2424) (-37.4001, 80.2528) (-37.4405, 80.2636) (-37.4808, 80.2746) (-37.5249, 80.2868) (-37.5688, 80.2993) (-37.6127, 80.3122) (-37.6603, 80.3262) (-37.7077, 80.3406) (-37.755, 80.3555) (-37.8061, 80.3715) (-37.8569, 80.3879) (-37.9077, 80.4048) (-37.9621, 80.423) (-38.0163, 80.4416) (-38.0704, 80.4607) (-38.1282, 80.4811) (-38.1858, 80.502) (-38.2431, 80.5234) (-38.3042, 80.5462) (-38.365, 80.5696) (-38.4256, 80.5934) (-38.4898, 80.6187) (-38.5538, 80.6446) (-38.6176, 80.671) (-38.6849, 80.6989) (-38.752, 80.7274) (-38.8189, 80.7565) (-38.9425, 80.8103) (-39.0653, 80.8661) (-39.1873, 80.9237) knots 0 0 0 0 0.057795 0.057795 0.057795 0.089038 0.089038 0.089038 0.118617 0.118617 0.118617 0.14653 0.14653 0.14653 0.172778 0.172778 0.172778 0.19736 0.19736 0.19736 0.220277 0.220277 0.220277 0.241529 0.241529 0.241529 0.261115 0.261115 0.261115 0.279036 0.279036 0.279036 0.295292 0.295292 0.295292 0.309882 0.309882 0.309882 0.329164 0.329164 0.329164 0.333477 0.333477 0.333477 0.337694 0.337694 0.337694 0.34182 0.34182 0.34182 0.345864 0.345864 0.345864 0.349834 0.349834 0.349834 0.353742 0.353742 0.353742 0.3576 0.3576 0.3576 0.361424 0.361424 0.361424 0.365232 0.365232 0.365232 0.369048 0.369048 0.369048 0.372899 0.372899 0.372899 0.376819 0.376819 0.376819 0.380853 0.380853 0.380853 0.385052 0.385052 0.385052 0.389482 0.389482 0.389482 0.394225 0.394225 0.394225 0.399381 0.399381 0.399381 0.405067 0.405067 0.405067 0.411413 0.411413 0.411413 0.418548 0.418548 0.418548 0.426565 0.426565 0.426565 0.435472 0.435472 0.435472 0.445133 0.445133 0.445133 0.45436 0.45436 0.45436 0.5 0.5 0.5 0.54564 0.54564 0.54564 0.554867 0.554867 0.554867 0.564528 0.564528 0.564528 0.573435 0.573435 0.573435 0.581452 0.581452 0.581452 0.588587 0.588587 0.588587 0.594933 0.594933 0.594933 0.600619 0.600619 0.600619 0.605775 0.605775 0.605775 0.610518 0.610518 0.610518 0.614948 0.614948 0.614948 0.619147 0.619147 0.619147 0.623181 0.623181 0.623181 0.627101 0.627101 0.627101 0.630952 0.630952 0.630952 0.634768 0.634768 0.634768 0.638576 0.638576 0.638576 0.6424 0.6424 0.6424 0.646258 0.646258 0.646258 0.650166 0.650166 0.650166 0.654136 0.654136 0.654136 0.65818 0.65818 0.65818 0.662306 0.662306 0.662306 0.666523 0.666523 0.666523 0.670836 0.670836 0.670836 0.690118 0.690118 0.690118 0.704708 0.704708 0.704708 0.720964 0.720964 0.720964 0.738885 0.738885 0.738885 0.758471 0.758471 0.758471 0.779723 0.779723 0.779723 0.80264 0.80264 0.80264 0.827222 0.827222 0.827222 0.85347 0.85347 0.85347 0.881383 0.881383 0.881383 0.910962 0.910962 0.910962 0.942205 0.942205 0.942205 1 1 1 1
  arc A226 (-39.325, 77.9647) -> (-39.3182, 76.8049) centre (0.0435, 77.6158) ccw